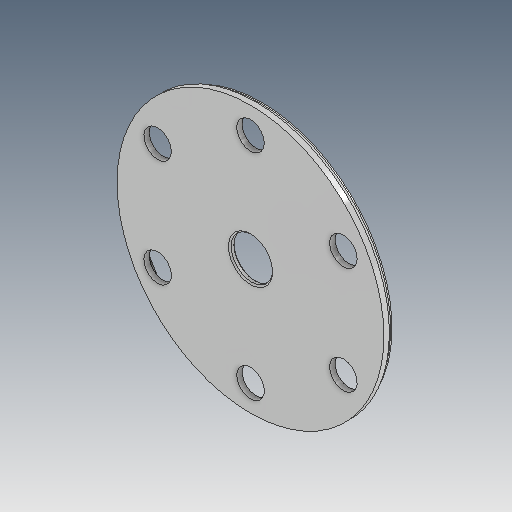
# Autodesk Inventor part: Front cover of servo motor
Saved by Autodesk Inventor 2020.3 (Build 243373010, 373A)
## iProperties
Created: 2021-04-08
Part Number: Front cover of servo motor
Material: Aluminum 6061-AHC
Document SubType Name: Modeling
Designer: marti
Density: 2.7 g/cm^3
Appearance: Aluminum - Dark
Mass: 4.91301 g
Surface Area: 38.7446 cm^2
Volume: 1.81963 cm^3
Author: marti
Autodesk Inventor part; units mm, degrees
ref_plane "YZ Plane" through (0, 0, 0) normal (1, 0, 0) x (0, 1, 0)
ref_plane "XZ Plane" through (0, 0, 0) normal (0, 1, 0) x (-1, 0, 0)
ref_plane "XY Plane" through (0, 0, 0) normal (0, 0, 1) x (1, 0, 0)
sketch "Sketch2" plane through (0, 0, 0) normal (1, 0, 0) x (0, 1, 0)
  line L0 (13.4931, 0) -> (24.25, 0)
  line L1 (24.25, 0) -> (24.25, -1)
  line L2 (24.25, -1) -> (23.7248, -1.75)
  line L3 (23.7248, -1.75) -> (23.7248, -2)
  line L4 (23.7248, -2) -> (23, -2)
  line L5 (0, 0) -> (0, -8.2884)
  line L6 (23, -2) -> (23, -1)
  line L7 (23, -1) -> (3.7625, -1)
  line L8 (13.4931, 0) -> (3.7625, 0)
  line L9 (3.7625, 0) -> (3.7625, -1)
  dimension "d3" = 1
  dimension "d4" = 145
  dimension "d5" = 0.75
  dimension "d7" = 0.25
  dimension "d8" = 2
  dimension "d10" = 48.5
  dimension "d11" = 47.4497
  dimension "d12" = 1.25
  dimension "d13" = 7.525
  constraints: 20 end point, 4 perpendicular, 4 vertical, 1 coincident, 1 horizontal
  measures "d3" distance of L0.end L1.end
  measures "d4" angle of L1 L2
  measures "d5" vertical distance of L1.end L2.end
  measures "d7" distance of L2.end L3.end
  measures "d8" distance between parallel lines of L0 L4
  measures "d10" diameter of L1 L5
  measures "d11" diameter of L3 L5
  measures "d12" distance between parallel lines of L1 L6
  measures "d13" diameter of L9 L5
revolve "Revolution1" add sketch "Sketch2" angle 360 about axis through (0, 0, 0) along (0, 0, -1)
sketch "Sketch3" plane through (0, 0, 0) normal (0, 0, 1) x (1, 0, 0)
  circle A0 centre (0, 0) radius 3.7625 projected
  circle A1 centre (0, 0) radius 3.7625 projected
  circle A2 centre (0, 0) radius 24.25 projected
  point P0 (0, 0)
  point P1 (0, 0)
  point P2 (0, 19.5)
  dimension "d15" = 19.5
  dimension "d16" = 48.5
  constraints: 1 coincident
  measures "d15" distance of point (0, 19.5) point (0, 0)
  measures "d16" diameter of A2
hole "Hole1" at (0, 0, 0) at (0, 19.5, 0) direction (0, 0, -1) diameter 5 end through all
pattern_circular "Circular Pattern1" count 6 over 360 about axis through (0, 0, -10) along (0, 0, 1) of "Hole1"
chamfer "Chamfer1" distance 0.25 angle 45 2 edges at (0, -3.7625, 0) (0, -3.7625, -1)
body "Solid2"
